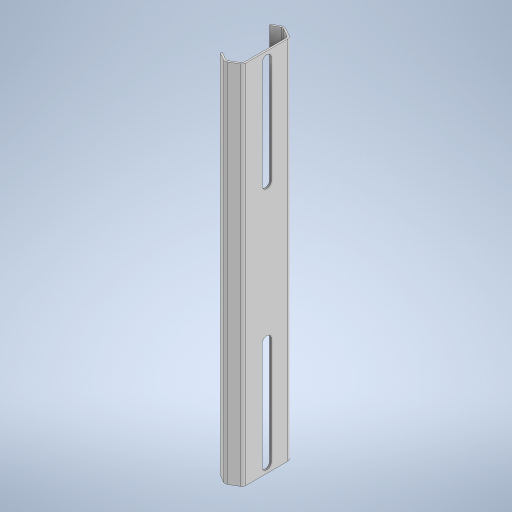
# Autodesk Inventor part: PoleBracket
Saved by Autodesk Inventor 2024.2 (Build 282272000, 272)
## iProperties
Created: 2024-01-15
Part Number: PoleBracket
Material: Generic
Document SubType Name: Modeling
Designer: airso
Density: 1 g/cm^3
Appearance: Default
Author: airso
Autodesk Inventor part; units mm, degrees
ref_plane "YZ Plane" through (0, 0, 0) normal (1, 0, 0) x (0, 1, 0)
ref_plane "XZ Plane" through (0, 0, 0) normal (0, 1, 0) x (-1, 0, 0)
ref_plane "XY Plane" through (0, 0, 0) normal (0, 0, 1) x (1, 0, 0)
sketch "Sketch1" plane through (0, 0, 0) normal (0, 1, 0) x (-1, 0, 0)
  line L0 (-17.018, 36.3476) -> (-17.018, 3.1529)
  line L1 (-15.4305, 0.4033) -> (-8.9535, -3.3362)
  line L2 (-5.7785, -3.3362) -> (0, 0)
  line L3 (-15.4305, 39.0972) -> (-8.9535, 42.8367)
  line L4 (-5.7785, 42.8367) -> (0, 39.5005)
  arc A0 (-15.4305, 39.0972) -> (-17.018, 36.3476) centre (-13.843, 36.3476) ccw
  arc A1 (-5.7785, 42.8367) -> (-8.9535, 42.8367) centre (-7.366, 40.0871) ccw
  arc A2 (-8.9535, -3.3362) -> (-5.7785, -3.3362) centre (-7.366, -0.5866) ccw
  arc A3 (-17.018, 3.1529) -> (-15.4305, 0.4033) centre (-13.843, 3.1529) ccw
  line L5 (-0.635, 1.0999) -> (-6.4135, -2.2364)
  arc A4 (-8.3185, -2.2364) -> (-6.4135, -2.2364) centre (-7.366, -0.5866) ccw
  line L6 (-8.3185, -2.2364) -> (-14.7955, 1.5031)
  arc A5 (-15.748, 3.1529) -> (-14.7955, 1.5031) centre (-13.843, 3.1529) ccw
  line L7 (-15.748, 3.1529) -> (-15.748, 36.3476)
  arc A6 (-14.7955, 37.9973) -> (-15.748, 36.3476) centre (-13.843, 36.3476) ccw
  line L8 (-14.7955, 37.9973) -> (-8.3185, 41.7368)
  arc A7 (-6.4135, 41.7368) -> (-8.3185, 41.7368) centre (-7.366, 40.0871) ccw
  line L9 (-6.4135, 41.7368) -> (-0.635, 38.4006)
  line L10 (0, 39.5005) -> (-0.635, 38.4006)
  line L11 (-0.635, 1.0999) -> (0, 0)
  point P0 (-17.018, 38.1807)
  point P1 (-17.018, 1.3198)
  point P2 (-7.366, -4.2528)
  point P3 (-7.366, 43.7532)
  dimension "d2" = 48.006
  dimension "d3" = 17.018
  dimension "d4" = 17.018
  dimension "d5" = 120
  dimension "d6" = 120
  dimension "d7" = 120
  dimension "d8" = 120
  dimension "d9" = 9.652
  dimension "d10" = 9.652
  dimension "d11" = 3.175
  dimension "d12" = 1.27
  constraints: 24 end point, 16 point on circle, 9 point on line, 8 centre point, 8 tangent, 3 equal radius, 1 perpendicular, 1 vertical, 8 other
  measures "d2" distance of point (-7.366, -4.253) point (-7.366, 43.753)
  measures "d3" horizontal distance of point (-17.018, 38.181) L4.end
  measures "d4" horizontal distance of point (-17.018, 1.32) L2.end
  measures "d5" angle of L0 L3
  measures "d6" angle of L0 L1
  measures "d7" angle of L3 L4
  measures "d8" angle of L1 L2
  measures "d9" horizontal distance of point (-17.018, 38.181) point (-7.366, 43.753)
  measures "d10" horizontal distance of point (-17.018, 1.32) point (-7.366, -4.253)
  measures "d11" radius of A0
  measures "d12" distance between parallel lines of L0 L7
extrude "Extrusion1" add sketch "Sketch1" along normal blind 290.068
sketch "Sketch2" plane through (15.748, 0, 3.1529) normal (-1, 0, 0) x (0, 0, 1)
  line L0 (13.0392, 6.096) -> (13.0392, 90.932)
  line L1 (20.1512, 6.096) -> (20.1512, 90.932)
  arc A0 (20.1512, 90.932) -> (13.0392, 90.932) centre (16.5952, 90.932) ccw
  arc A1 (13.0392, 6.096) -> (20.1512, 6.096) centre (16.5952, 6.096) ccw
  line L2 (13.0392, 199.136) -> (13.0392, 283.972)
  line L3 (20.1512, 199.136) -> (20.1512, 283.972)
  arc A2 (20.1512, 283.972) -> (13.0392, 283.972) centre (16.5952, 283.972) ccw
  arc A3 (13.0392, 199.136) -> (20.1512, 199.136) centre (16.5952, 199.136) ccw
  line L4 (0, 0) -> (33.1947, 0) projected
  line L5 (39.6838, 0) -> (39.6838, 290.068) projected
  point P0 (-3.1529, 0)
  point P1 (16.5952, 94.488)
  point P2 (16.5952, 2.54)
  point P3 (16.5952, 94.488)
  point P4 (16.5952, 195.58)
  point P5 (16.5952, 287.528)
  dimension "d16" = 101.092
  dimension "d17" = 91.948
  dimension "d18" = 91.948
  dimension "d19" = 2.54
  dimension "d20" = 23.0886
  dimension "d21" = 23.0886
  dimension "d22" = 7.112
  dimension "d23" = 7.112
  constraints: 13 point on circle, 8 end point, 8 tangent, 4 centre point, 4 vertical
  measures "d16" distance of point (16.595, 195.58) point (16.595, 94.488)
  measures "d17" distance of point (16.595, 94.488) point (16.595, 2.54)
  measures "d18" distance of point (16.595, 287.528) point (16.595, 195.58)
  measures "d19" distance from line of point (16.595, 2.54) L4
  measures "d20" distance from line of L5 A1.centre
  measures "d21" distance from line of L5 A3.centre
  measures "d22" distance between parallel lines of L1 L0
  measures "d23" distance between parallel lines of L3 L2
extrude "Extrusion2" cut sketch "Sketch2" against normal through all
body "Solid1"
